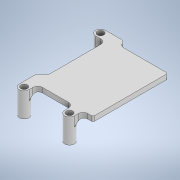
# Autodesk Inventor part: BreadboardPlate
Saved by Autodesk Inventor 2020 (Build 240168000, 168)
## iProperties
Created: 2019-04-20
Part Number: BreadboardPlate
Material: Generic
Document SubType Name: Modeling
Designer: mfans
Density: 1 g/cm^3
Appearance: Default
Author: mfans
Autodesk Inventor part; units mm, degrees
ref_plane "YZ Plane" through (0, 0, 0) normal (1, 0, 0) x (0, 1, 0)
ref_plane "XZ Plane" through (0, 0, 0) normal (0, 1, 0) x (-1, 0, 0)
ref_plane "XY Plane" through (0, 0, 0) normal (0, 0, 1) x (1, 0, 0)
sketch "Sketch1" plane through (0, 0, 0) normal (0, 1, 0) x (-1, 0, 0)
  line L0 (18, -23) -> (-18, -23)
  line L1 (-18, -23) -> (-18, 23)
  line L2 (-18, 23) -> (18, 23)
  line L3 (18, 23) -> (18, -23)
  line L4 (18, -23) -> (-18, 23) construction
  line L5 (-18, -23) -> (18, 23) construction
  circle A0 centre (19, 28.3696) radius 3
  circle A1 centre (-8.9, 28.3696) radius 3
  circle A2 centre (24.1, -23.7304) radius 3
  line L6 (24.1, -26.7304) -> (12.1, -26.7304)
  line L7 (12.1, -26.7304) -> (12.1, -20.7304)
  line L8 (12.1, -20.7304) -> (24.1, -20.7304)
  line L9 (24.1, -20.7304) -> (24.1, -26.7304)
  line L10 (-5.9, 28.3696) -> (-11.9, 28.3696)
  line L11 (-11.9, 28.3696) -> (-11.9, 23)
  line L12 (-11.9, 23) -> (-5.9, 23)
  line L13 (-5.9, 23) -> (-5.9, 28.3696)
  line L14 (22, 28.3696) -> (16, 28.3696)
  line L15 (16, 28.3696) -> (16, 16.3696)
  line L16 (16, 16.3696) -> (22, 16.3696)
  line L17 (22, 16.3696) -> (22, 28.3696)
  point P0 (0, 0)
  point P1 (-24.1, -22.4304)
  point P2 (16, 23)
  point P3 (12.1, -23)
  point P4 (18, -20.7304)
  point P5 (18, 16.3696)
  dimension "d12" = 6
  dimension "d13" = 6
  dimension "d14" = 6
  dimension "d0" = 46
  dimension "d1" = 36
  dimension "d6" = 27.9
  dimension "d7" = 15.2
  dimension "d8" = 5.1
  dimension "d9" = 1.3
  dimension "d10" = 50.8
  dimension "d11" = 6.1
  dimension "d15" = 12
  dimension "d16" = 12
  constraints: 36 end point, 8 parallel, 4 horizontal, 4 perpendicular, 3 coincident, 2 midpoint, 1 point on line, 9 other
  measures "d0" distance of L0.end L1.end
  measures "d1" distance of L0.start L0.end
  measures "d6" distance of point (-8.9, 28.37) point (19, 28.37)
  measures "d7" horizontal distance of point (-24.1, -22.43) point (-8.9, 28.37)
  measures "d8" horizontal distance of point (19, 28.37) point (24.1, -23.73)
  measures "d9" vertical distance of point (24.1, -23.73) point (-24.1, -22.43)
  measures "d10" vertical distance of point (-8.9, 28.37) point (-24.1, -22.43)
  measures "d11" distance from line of L1 point (-24.1, -22.43)
  measures "d15" distance of L6.start L6.end
  measures "d16" distance of L16.end L14.start
extrude "Extrusion1" add sketch "Sketch1" along normal blind 3
fillet "Fillet1" radius 3 8 edges at (-12.1, 1.5, -26.7304) (-12.1, 1.5, -23) (-18, 1.5, -20.7304) (-18, 1.5, 16.3696) (-22, 1.5, 16.3696) (-16, 1.5, 23) (5.9, 1.5, 23) (11.9, 1.5, 23)
sketch "Sketch2" plane through (0, 0, 0) normal (0, -1, 0) x (1, 0, 0)
  arc A0 (-14.6542, -26.7304) -> (-11.8771, -24.8652) centre (-14.6542, -23.7304) ccw projected
  arc A1 (-9.1, -23) -> (-11.8771, -24.8652) centre (-9.1, -26) ccw projected
  line L0 (18, -23) -> (-9.1, -23) projected
  line L1 (18, 23) -> (18, -23) projected
  line L2 (14.9, 23) -> (18, 23) projected
  arc A2 (11.9, 26) -> (14.9, 23) centre (14.9, 26) ccw projected
  line L3 (11.9, 28.3696) -> (11.9, 26) projected
  arc A3 (11.9, 28.3696) -> (5.9, 28.3696) centre (8.9, 28.3696) ccw projected
  line L4 (5.9, 26) -> (5.9, 28.3696) projected
  arc A4 (2.9, 23) -> (5.9, 26) centre (2.9, 26) ccw projected
  line L5 (-13, 23) -> (2.9, 23) projected
  arc A5 (-16, 26) -> (-13, 23) centre (-13, 26) ccw projected
  line L6 (-16, 28.3696) -> (-16, 26) projected
  arc A6 (-16, 28.3696) -> (-22, 28.3696) centre (-19, 28.3696) ccw projected
  line L7 (-22, 19.0264) -> (-22, 28.3696) projected
  arc A7 (-22, 19.0264) -> (-20, 16.198) centre (-19, 19.0264) ccw projected
  arc A8 (-18, 13.3696) -> (-20, 16.198) centre (-21, 13.3696) ccw projected
  line L8 (-18, -17.7304) -> (-18, 13.3696) projected
  arc A9 (-21, -20.7304) -> (-18, -17.7304) centre (-21, -17.7304) ccw projected
  line L9 (-24.1, -20.7304) -> (-21, -20.7304) projected
  arc A10 (-24.1, -20.7304) -> (-24.1, -26.7304) centre (-24.1, -23.7304) ccw projected
  line L10 (-14.6542, -26.7304) -> (-24.1, -26.7304) projected
  circle A11 centre (-19, 28.3696) radius 3
  circle A12 centre (8.9, 28.3696) radius 3
  circle A13 centre (-24.1, -23.7304) radius 3
  point P0 (0, 0)
  constraints: 3 coincident, 2 centre point, 2 concentric, 3 other
extrude "Extrusion2" add sketch "Sketch2" along normal blind 12 contours A10 A13 | A12 A3 | A6 A11
fillet "Fillet2" radius 3 3 edges at (-21.1, 0, -23.7304) (-19, 0, 25.3696) (8.9, 0, 25.3696)
sketch "Sketch3" plane through (0, 3, 0) normal (0, 1, 0) x (1, 0, 0)
  arc A0 (-11.8771, 24.8652) -> (-14.6542, 26.7304) centre (-14.6542, 23.7304) ccw projected
  line L0 (-14.6542, 26.7304) -> (-24.1, 26.7304) projected
  arc A1 (-24.1, 26.7304) -> (-24.1, 20.7304) centre (-24.1, 23.7304) ccw projected
  line L1 (-24.1, 20.7304) -> (-21, 20.7304) projected
  arc A2 (-18, 17.7304) -> (-21, 20.7304) centre (-21, 17.7304) ccw projected
  line L2 (-18, 17.7304) -> (-18, -13.3696) projected
  arc A3 (-20, -16.198) -> (-18, -13.3696) centre (-21, -13.3696) ccw projected
  arc A4 (-20, -16.198) -> (-22, -19.0264) centre (-19, -19.0264) ccw projected
  line L3 (-22, -19.0264) -> (-22, -28.3696) projected
  arc A5 (-22, -28.3696) -> (-16, -28.3696) centre (-19, -28.3696) ccw projected
  line L4 (-16, -28.3696) -> (-16, -26) projected
  arc A6 (-13, -23) -> (-16, -26) centre (-13, -26) ccw projected
  line L5 (-13, -23) -> (2.9, -23) projected
  arc A7 (5.9, -26) -> (2.9, -23) centre (2.9, -26) ccw projected
  line L6 (5.9, -26) -> (5.9, -28.3696) projected
  arc A8 (5.9, -28.3696) -> (11.9, -28.3696) centre (8.9, -28.3696) ccw projected
  line L7 (11.9, -28.3696) -> (11.9, -26) projected
  arc A9 (14.9, -23) -> (11.9, -26) centre (14.9, -26) ccw projected
  line L8 (14.9, -23) -> (18, -23) projected
  line L9 (18, -23) -> (18, 23) projected
  line L10 (18, 23) -> (-9.1, 23) projected
  arc A10 (-11.8771, 24.8652) -> (-9.1, 23) centre (-9.1, 26) ccw projected
  point P0 (0, 0)
  constraints: 3 coincident
hole "Hole1" at (-24.1, 3, -23.7304) at (8.9, 3, 28.3696) at (-19, 3, 28.3696) direction (0, -1, 0) diameter 4 end through all
fillet "Fillet3" radius 1 2 edges at (18, 1.5, -23) (18, 1.5, 23)
body "Solid1"
